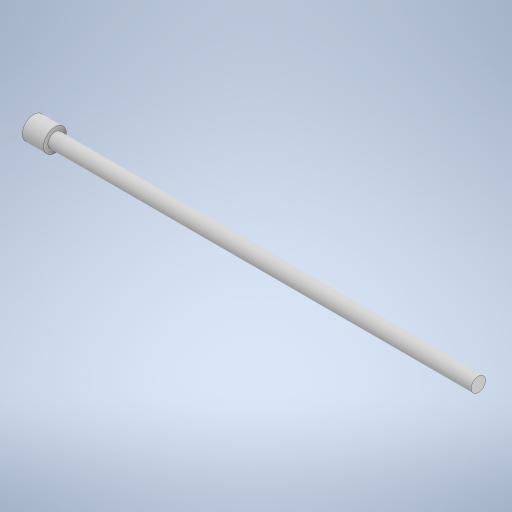
# Autodesk Inventor part: wormgear_axis_6mm
Saved by Autodesk Inventor 2024 (Build 280153000, 153)
## iProperties
Created: 2025-12-09
Part Number: wormgear_axis_6mm
Material: Generic
Document SubType Name: Modeling
Designer: schar
Density: 1 g/cm^3
Appearance: Default
Author: schar
Autodesk Inventor part; units mm, degrees
ref_plane "YZ Plane" through (0, 0, 0) normal (1, 0, 0) x (0, 1, 0)
ref_plane "XZ Plane" through (0, 0, 0) normal (0, 1, 0) x (-1, 0, 0)
ref_plane "XY Plane" through (0, 0, 0) normal (0, 0, 1) x (1, 0, 0)
sketch "Sketch1" plane through (0, 0, 0) normal (1, 0, 0) x (0, 1, 0)
  circle A0 centre (0, 0) radius 4
  circle A1 centre (0, 0) radius 2.5
  line L0 (2, 0) -> (2, -1.5)
  line L1 (2, 0) -> (2, 1.5)
  dimension "d0" = 8
  dimension "d1" = 5
  constraints: 4 end point, 2 centre point, 2 coincident, 2 point on circle, 1 point on line
  measures "d0" diameter of A0
  measures "d1" diameter of A1
extrude "Extrusion1" add sketch "Sketch1" along normal blind 8 contours A0 | A1 L0 L1 picked at (2.0912, -0.8466)
sketch "Sketch2" plane through (8, 0, 0) normal (1, 0, 0) x (0, 0, -1)
  circle A0 centre (0, 0) radius 4
  circle A1 centre (0, 0) radius 2.5
  constraints: 2 centre point, 2 coincident
extrude "Extrusion2" add sketch "Sketch2" along normal blind 2
sketch "Sketch3" plane through (8, 0, 0) normal (1, 0, 0) x (0, 0, -1)
  circle A0 centre (0, 0) radius 2.5
  constraints: 1 centre point, 1 coincident
extrude "Extrusion3" add sketch "Sketch3" along normal blind 151
sketch "Sketch4" plane through (0, 0, 0) normal (-1, 0, 0) x (0, 0, 1)
  circle A0 centre (0, 0) radius 4
  constraints: 1 centre point, 1 coincident
extrude "Extrusion4" cut sketch "Sketch4" against normal blind 2.5
sketch "Sketch5" plane through (0, 0, 0) normal (0, 1, 0) x (-1, 0, 0)
  line L0 (-152.0201, 0) -> (-91.0201, 0)
  line L1 (-91.0201, 0) -> (-90.0201, 0)
  circle A0 centre (-90.0201, 0) radius 1
  point P0 (0, 0)
  dimension "d11" = 61
  dimension "d12" = 1
  constraints: 4 end point, 1 coincident, 1 horizontal, 1 horizontal alignment, 1 point on line, 2 other
  measures "d11" distance of L0.start L0.end
  measures "d12" distance of L0.end L1.end
extrude "Extrusion5" cut sketch "Sketch5" against normal blind 10
thread "Thread1" size "M2x0.4" class "6H" standard "ANSI Metric M Profile" full length
body "Solid1"
